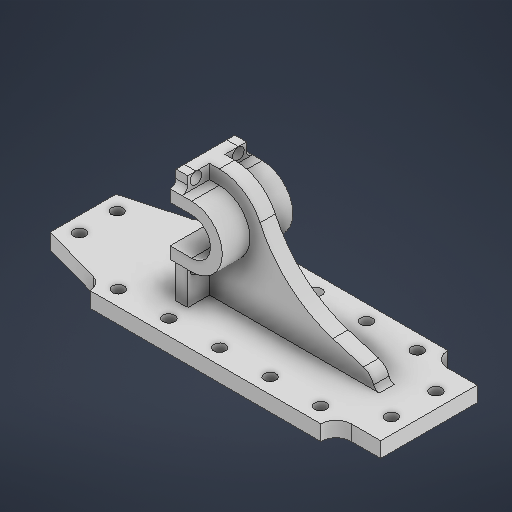
# Autodesk Inventor part: b9
Saved by Autodesk Inventor 2025.4 (Build 294407000, 407)
## iProperties
Created: 2026-05-15
Part Number: b9
Material: Generic
Document SubType Name: Modeling
Designer: VuQuan
Density: 1 g/cm^3
Appearance: Default
Author: VuQuan
Autodesk Inventor part; units mm, degrees
ref_plane "YZ Plane" through (0, 0, 0) normal (1, 0, 0) x (0, 1, 0)
ref_plane "XZ Plane" through (0, 0, 0) normal (0, 1, 0) x (-1, 0, 0)
ref_plane "XY Plane" through (0, 0, 0) normal (0, 0, 1) x (1, 0, 0)
sketch "Sketch1" plane through (0, 0, 0) normal (0, 1, 0) x (-1, 0, 0)
  line L0 (147, 0) -> (-147, 0) construction
  line L1 (147, 0) -> (147, -28)
  line L2 (147, -28) -> (96.5152, -42.0007)
  arc A0 (96.5152, -42.0007) -> (87, -54) centre (99.9893, -54.5279) ccw
  line L3 (87, -54) -> (-109, -54)
  arc A1 (-109, -54) -> (-122, -41) centre (-122, -54) ccw
  line L4 (-122, -41) -> (-147, -41)
  line L5 (-147, -41) -> (-147, 0)
  line L6 (147, 0) -> (147, 28)
  line L7 (147, 28) -> (96.5152, 42.0007)
  arc A2 (87, 54) -> (96.5152, 42.0007) centre (99.9893, 54.5279) ccw
  line L8 (87, 54) -> (-109, 54)
  arc A3 (-122, 41) -> (-109, 54) centre (-122, 54) ccw
  line L9 (-122, 41) -> (-147, 41)
  line L10 (-147, 41) -> (-147, 0)
  circle A4 centre (134, -16) radius 5
  circle A5 centre (-134, -19) radius 5
  circle A6 centre (-96, -41) radius 5
  circle A7 centre (-53, -41) radius 5
  circle A8 centre (-10, -41) radius 5
  circle A9 centre (33, -41) radius 5
  circle A10 centre (76, -41) radius 5
  circle A11 centre (134, 16) radius 5
  circle A12 centre (-134, 19) radius 5
  circle A13 centre (-96, 41) radius 5
  circle A14 centre (-53, 41) radius 5
  circle A15 centre (-10, 41) radius 5
  circle A16 centre (33, 41) radius 5
  circle A17 centre (76, 41) radius 5
  point P0 (0, 0)
  point P1 (0, 0)
  dimension "d0" = 56
  dimension "d1" = 294
  dimension "d2" = 82
  dimension "d3" = 196
  dimension "d5" = 38
  dimension "d6" = 108
  dimension "d7" = 13
  dimension "d8" = 10
  dimension "d9" = 13
  dimension "d10" = 32
  dimension "d11" = 13
  dimension "d12" = 38
  dimension "d13" = 51
  dimension "d16" = 43
  dimension "d21" = 31
  constraints: 23 end point, 18 centre point, 15 symmetric about line, 8 point on circle, 3 equal radius, 3 horizontal, 2 tangent, 1 coincident, 1 midpoint, 1 parallel, 1 perpendicular, 1 point on line, 1 vertical, 17 other
  measures "d0" diameter of L1.end L0
  measures "d1" distance of L0.start L0.end
  measures "d2" diameter of L4 L0
  measures "d3" distance of L3.start L3.end
  measures "d5" distance from line of L5 L3.end
  measures "d6" diameter of L3 L0
  measures "d7" radius of A0
  measures "d8" diameter of A4
  measures "d9" distance from line of L1 A4.centre
  measures "d10" diameter of A4.centre L0
  measures "d11" distance from line of L5 A5.centre
  measures "d12" diameter of A5.centre L0
  measures "d13" distance from line of L5 A6.centre
  measures "d16" distance of A6.centre A7.centre
  measures "d21" angle of L2 L7
extrude "Extrusion1" add sketch "Sketch1" along normal blind 13
sketch "Sketch2" plane through (0, 0, 0) normal (0, 0, 1) x (1, 0, 0)
  line L0 (-96.5152, 13) -> (-87, 13) projected
  line L1 (-87, 13) -> (109, 13) projected
  line L2 (109, 13) -> (122, 13) projected
  line L3 (122, 13) -> (147, 13) projected
  line L4 (147, 13) -> (122, 13) projected
  line L5 (122, 13) -> (109, 13) projected
  line L6 (109, 13) -> (-87, 13) projected
  line L7 (-87, 13) -> (-96.5152, 13) projected
  line L8 (-96.5152, 13) -> (-147, 13) projected
  line L9 (-147, 13) -> (-96.5152, 13) projected
  line L10 (91, 13) -> (101, 13) projected
  line L11 (-38, 13) -> (-28, 13) projected
  line L12 (48, 13) -> (58, 13) projected
  line L13 (-139, 13) -> (-129, 13) projected
  line L14 (-81, 13) -> (-71, 13) projected
  line L15 (-38, 13) -> (-28, 13) projected
  line L16 (5, 13) -> (15, 13) projected
  line L17 (48, 13) -> (58, 13) projected
  line L18 (91, 13) -> (101, 13) projected
  line L19 (129, 13) -> (139, 13) projected
  line L20 (-139, 13) -> (-129, 13) projected
  line L21 (129, 13) -> (139, 13) projected
  line L22 (5, 13) -> (15, 13) projected
  line L23 (-81, 13) -> (-71, 13) projected
  arc A0 (106.4884, 16.6111) -> (111.2916, 13) centre (111.2916, 18) ccw
  arc A1 (106.4884, 16.6111) -> (97.7907, 25.435) centre (94, 13) ccw
  arc A2 (9.9289, 87.6957) -> (71.8404, 33.3458) centre (101, 129) ccw
  arc A3 (9.9289, 87.6957) -> (-24.6782, 110) centre (-24.6782, 72) ccw
  line L24 (97.7907, 25.435) -> (71.8404, 33.3458)
  line L25 (-87, 13) -> (109, 13) projected
  line L26 (-43, 13) -> (-43, 56)
  line L27 (-43, 88) -> (-43, 110)
  line L28 (-24.6782, 110) -> (-43, 110)
  line L29 (-33, 13) -> (-33, 46)
  line L30 (-33, 98) -> (-33, 110)
  line L31 (-43, 56) -> (-24.6782, 56)
  arc A4 (-24.6782, 56) -> (-24.6782, 88) centre (-24.6782, 72) ccw
  line L32 (-24.6782, 88) -> (-43, 88)
  line L33 (-33, 46) -> (-24.6782, 46)
  arc A5 (-24.6782, 46) -> (-24.6782, 98) centre (-24.6782, 72) ccw
  line L34 (-24.6782, 98) -> (-33, 98)
  point P0 (0, 0)
  dimension "d24" = 5
  dimension "d25" = 13
  dimension "d26" = 53
  dimension "d27" = 100
  dimension "d29" = 46
  dimension "d30" = 38
  dimension "d32" = 116
  dimension "d33" = 190
  dimension "d36" = 10
  dimension "d37" = 16
  dimension "d38" = 26
  dimension "d39" = 59
  constraints: 20 end point, 12 point on circle, 10 tangent, 6 centre point, 5 horizontal, 4 point on line, 2 coincident, 2 collinear, 2 vertical, 1 parallel, 3 other
  measures "d24" radius of A0
  measures "d25" radius of A1
  measures "d26" distance of L3.end A1.centre
  measures "d27" radius of A2
  measures "d29" horizontal distance of L3.end A2.centre
  measures "d30" radius of A3
  measures "d32" distance from line of L1 A2.centre
  measures "d33" distance of L3.end L26.start
  measures "d36" distance between parallel lines of L26 L29
  measures "d37" radius of A4
  measures "d38" radius of A5
  measures "d39" distance from line of A5.centre L1
extrude "Extrusion2" add sketch "Sketch2" along normal mid plane 60 contours L26 L31 A4 L32 L27 L28 L30 L34 A5 L33 L29 L1
extrude "Rib1" add sketch "Sketch2" along normal mid plane 13 rib yes fills toward (-42.95, 34.5) open curves L26 L31 A4 L32 L27 L28 A3 A2 L24 A1 A0
sketch "Sketch3" plane through (-43, 13, -30) normal (-1, 0, 0) x (0, 0, 1)
  line L0 (0, 0) -> (0, 43) projected
  line L1 (60, 0) -> (0, 0) projected
  line L2 (60, 43) -> (60, 0) projected
  line L3 (0, 97) -> (23.5, 97) projected
  line L4 (5, 97) -> (5, 90)
  arc A0 (0, 85) -> (5, 90) centre (0, 90) ccw
  line L5 (0, 75) -> (0, 97) projected
  line L6 (30, 0) -> (30, 97) construction
  line L7 (36.5, 97) -> (23.5, 97) projected
  line L8 (0, 43) -> (0, 75) projected
  line L9 (60, 75) -> (60, 43) projected
  line L10 (0, 59) -> (60, 59) construction
  line L11 (55, 97) -> (55, 90)
  arc A1 (55, 90) -> (60, 85) centre (60, 90) ccw
  line L12 (5, 0) -> (5, 28)
  arc A2 (5, 28) -> (0, 33) centre (0, 28) ccw
  line L13 (55, 0) -> (55, 28)
  arc A3 (60, 33) -> (55, 28) centre (60, 28) ccw
  line L14 (0, 97) -> (60, 97) projected
  line L15 (60, 97) -> (60, 75) projected
  point P0 (30, -13)
  point P1 (30, 59)
  point P2 (5, 21)
  point P3 (55, 21)
  dimension "d50" = 5
  dimension "d51" = 50
  constraints: 12 end point, 12 symmetric about line, 8 point on circle, 5 midpoint, 5 point on line, 4 centre point, 1 horizontal, 1 tangent, 1 vertical, 3 other
  measures "d50" radius of A0
  measures "d51" diameter of L4 L6
extrude "Extrusion3" cut sketch "Sketch3" against normal up to surface (10 mm away) contours L0 A2 L12 L1 | L13 A3 L2 L1 | L5 L3 L4 A0 | A1 L11 L14 L15
sketch "Sketch4" plane through (-43, 88, -30) normal (-1, 0, 0) x (0, 0, 1)
  line L0 (55, 15) -> (55, 22) projected
  line L1 (5, 22) -> (55, 22) projected
  circle A0 centre (48, 17) radius 5
  line L2 (22, -16) -> (38, -16) construction
  line L3 (30, -21) -> (30, -11) construction
  circle A1 centre (12, 17) radius 5
  circle A2 centre (48, -49) radius 5
  circle A3 centre (12, -49) radius 5
  point P0 (30, -88)
  point P1 (30, -16)
  dimension "d54" = 7
  dimension "d55" = 5
  dimension "d56" = 10
  constraints: 4 centre point, 4 end point, 3 midpoint, 3 symmetric about line, 1 horizontal, 1 vertical, 3 other
  measures "d54" distance from line of L0 A0.centre
  measures "d55" distance from line of L1 A0.centre
  measures "d56" diameter of A0
extrude "Extrusion4" cut sketch "Sketch4" against normal blind 10
body "Solid1"
